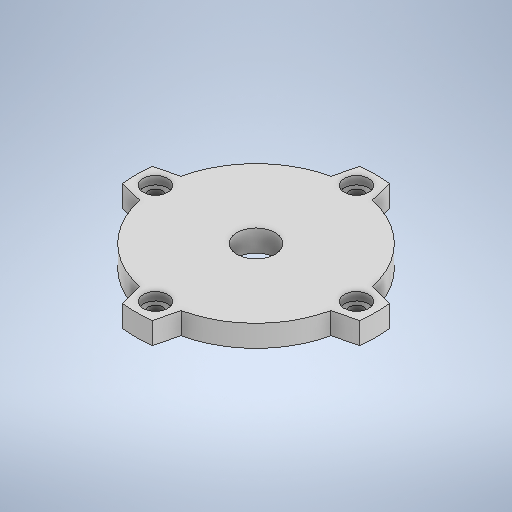
# Autodesk Inventor part: shaft_lock_2
Saved by Autodesk Inventor 2025 (Build 290162000, 162)
## iProperties
Created: 2026-08-04
Part Number: shaft_lock_2
Material: Ogólny
Document SubType Name: Modeling
Designer: zzapa
Density: 1 g/cm^3
Appearance: Domyślna
Author: zzapa
Autodesk Inventor part; units mm, degrees
ref_plane "YZ Plane" through (0, 0, 0) normal (1, 0, 0) x (0, 1, 0)
ref_plane "XZ Plane" through (0, 0, 0) normal (0, 1, 0) x (-1, 0, 0)
ref_plane "XY Plane" through (0, 0, 0) normal (0, 0, 1) x (1, 0, 0)
sketch "Szkic1" plane through (0, 0, 0) normal (0, 1, 0) x (-1, 0, 0)
  circle A0 centre (0, 0) radius 22
  circle A1 centre (0, 0) radius 3.5
  circle A2 centre (0, 0) radius 18
  line L0 (-17.5943, -3.8) -> (-21.8274, -2.75)
  line L1 (30.8, 0) -> (-30.8, 0) projected
  line L2 (-17.5943, 3.8) -> (-21.8274, 2.75)
  line L3 (3.8, -17.5943) -> (2.75, -21.8274)
  line L4 (-3.8, -17.5943) -> (-2.75, -21.8274)
  line L5 (17.5943, 3.8) -> (21.8274, 2.75)
  line L6 (17.5943, -3.8) -> (21.8274, -2.75)
  line L7 (-3.8, 17.5943) -> (-2.75, 21.8274)
  line L8 (3.8, 17.5943) -> (2.75, 21.8274)
  point P0 (17.5943, -3.8)
  point P1 (21.8274, -2.75)
  point P2 (21.8274, 2.75)
  point P3 (17.5943, 3.8)
  point P4 (2.75, 21.8274)
  point P5 (-2.75, 21.8274)
  point P6 (-3.8, 17.5943)
  point P7 (-17.5943, 3.8)
  point P8 (-21.8274, 2.75)
  point P9 (-3.8, -17.5943)
  point P10 (-2.75, -21.8274)
  point P11 (2.75, -21.8274)
  dimension "d1" = 44
  dimension "d2" = 36
  dimension "d0" = 7
  dimension "d3" = 5.5
  dimension "d4" = 7.6
  dimension "d7" = 360
  constraints: 16 end point, 3 coincident, 2 symmetric about line, 1 centre point, 31 other
  measures "d0" diameter of A1
  measures "d3" distance of L0.end L2.end
  measures "d4" distance of L2.start L0.start
extrude "Wyciągnięcie proste1" add sketch "Szkic1" along normal blind 4 contours L1 A2 L5 A0 | A0 L6 A2 L1 | L1 A1 A2 | A2 L1 A1 | L8 A2 L7 A0 | A0 L4 A2 L3 | L2 A2 L1 A0 | A0 L1 A2 L0
sketch "Szkic2" plane through (0, 4, 0) normal (0, 1, 0) x (1, 0, 0)
  line L0 (-30.8, 0) -> (30.8, 0) projected
  point P0 (0, 0)
  point P1 (18.5, 0)
  point P2 (0, 18.5)
  point P3 (-18.5, 0)
  point P4 (0, -18.5)
  dimension "d11" = 18.5
  dimension "d14" = 360
  constraints: 1 point on line, 5 other
  measures "d11" distance of point (0, 0) point (18.5, 0)
hole "Otwór1" at (18.5, 4, 0) at (0, 4, -18.5) at (-18.5, 4, 0) at (0, 4, 18.5) direction (0, -1, 0) diameter 2.6 end through all counterbore diameter 4.5 counterbore depth 1.5
equation "\"d1\" = shaft_lock_2_D"
equation "\"d2\" = shaft_lock_2_rotor_insert_grove_d_in"
equation "\"d0\" = shaft_lock_2_d"
equation "\"d3\" = shaft_lock_2_rotor_insert_grove_width_out"
equation "\"d4\" = shaft_lock_2_rotor_insert_grove_width_in"
equation "\"d9\" = shaft_lock_2_h1"
equation "\"d11\" = 0.5 * shaft_lock_2_rotor_insert_r"
equation "\"d16\" = insert_m2_pocket_d"
equation "\"d18\" = insert_m2_pocket_D"
equation "\"d19\" = insert_m2_pocket_nut_h"
equation "\"insert25m_d\" = 2.9"
equation "\"insert25m_h\" = 7"
equation "\"insert25m_corner\" = 0.5"
equation "\"stator_out_d\" = 2.5"
equation "\"stator_h\" = 35"
equation "\"mag_size_x\" = 7"
equation "\"mag_size_y\" = 3"
equation "\"mag_corner_r\" = 0.4"
equation "\"magnet_ring_r\" = 27.5"
equation "\"magnet_ring_d\" = 3.3"
equation "\"magnet_ring_h\" = 36"
equation "\"magnet_ring_pocket_mag_size_x\" = 7.1"
equation "\"magnet_ring_pocket_mag_size_y\" = 3.1"
equation "\"magnet_ring_pocket_mag_size_z\" = 10.3"
equation "\"magnet_ring_pocket_radial_cut\" = 1.4"
equation "\"casing_d\" = 3"
equation "\"rotor_out_r\" = 23"
equation "\"rotor_coil_groove_in_r\" = 17"
equation "\"rotor_coil_groove_ang\" = 18deg"
equation "\"rotor_core_r\" = 15"
equation "\"rotor_coil_groove_in_correction_r\" = 18"
equation "\"rotor_plastic_h\" = 32"
equation "\"rotor_teeth_d\" = 1.5"
equation "\"rotor_plastic_insert_r\" = 37"
equation "\"shaft_d\" = 8"
equation "\"shaft_lock_1_d\" = 8"
equation "\"shaft_lock_1_D\" = 36"
equation "\"shaft_lock_1_h1\" = 4"
equation "\"shaft_lock_1_corner\" = 1"
equation "\"shaft_lock_1_insert_part_h\" = 7"
equation "\"shaft_lock_1_insert_part_a\" = 18"
equation "\"shaft_lock_2_h1\" = 4"
equation "\"shaft_lock_2_d\" = 7"
equation "\"shaft_lock_2_insert_part_a\" = 18"
equation "\"shaft_lock_2_D\" = 44"
equation "\"shaft_lock_2_corner\" = 1"
equation "\"shaft_lock_2_insert_part_h\" = 7"
equation "\"shaft_lock_2_rotor_insert_grove_d_in\" = 36"
equation "\"shaft_lock_2_rotor_insert_grove_width_out\" = 5.5"
equation "\"shaft_lock_2_rotor_insert_grove_width_in\" = 7.6"
equation "\"shaft_lock_2_rotor_insert_r\" = 37"
equation "\"shaft_lock_2_rotor_insert_screw_d\" = 2.6"
equation "\"insert25m_pocket_d\" = 2.6"
equation "\"insert25m_pocket_D\" = 4.5"
equation "\"insert25m_pocket_nut_h\" = 1.5"
equation "\"insert_m2_pocket_d\" = 2.6"
equation "\"insert_m2_h\" = 7"
equation "\"insert_m2_d\" = 2.9"
equation "\"insert_m2_corner\" = 0.5"
equation "\"insert_m2_pocket_D\" = 4.5"
equation "\"insert_m2_pocket_nut_h\" = 1.5"
